Autodesk Fusion 360 part; units mm, degrees
(part 2 of 2)
sketch "Dovetail" plane through (75.5, 0, 0) normal (1, 0, 0) x (0, 1, 0)
  line L0 (-30.5, 0) -> (30.5, 0)
  line L1 (30.5, 0) -> (30.5, 32)
  line L2 (30.5, 32) -> (-30.5, 32)
  line L3 (-30.5, 32) -> (-30.5, 0)
  line L4 (-27.5, 32) -> (-27.5, 5.5)
  line L5 (-27.5, 5.5) -> (-27.5, 32)
  line L6 (27.5, 5.5) -> (27.5, 32)
  line L7 (27.5, 32) -> (27.5, 5.5)
  line L8 (30.5, 0) -> (30.5, 32)
  line L9 (-30.5, 0) -> (-30.5, 32)
  line L10 (-30.5, 29) -> (30.5, 29)
  line L11 (-28.9434, 29) -> (-27.5, 31.5)
  line L12 (-28.9434, 29) -> (-27.5, 29) construction
  line L13 (0, 2.5) -> (0, 20)
  line L14 (28.9434, 29) -> (27.5, 31.5)
  dimension "d19" = 3
  dimension "d20" = 60
  dimension "d21" = 0.5
  constraint coincident L9 L10.start
  constraint coincident L8 L10.end
  constraint perpendicular L8 L10
  constraint horizontal L12
  constraint coincident L10 L11.start
  constraint coincident L5 L11.end
  constraint symmetric L11.start L13 L14.start
  constraint symmetric L11.end L13 L14.end
  constraint coincident L4 L12.end
  measures "d19" distance of L2 L10
  measures "d20" angle of L11 L12
  measures "d21" distance of L2 L11.end
extrude "Extrude4" cut sketch "Dovetail" against normal up to surface (148 mm away) contours L4 L5 L10 L11 | L6 L7 L10 L14 | L2 L4 L5 L6 L7 L10 bodies 1
sketch "Lid" plane through (75.5, 0, 0) normal (1, 0, 0) x (0, 1, 0) in component "Lid"
  line L0 (27.5, 32) -> (27.5, 31.5)
  line L1 (27.5, 31.5) -> (28.9434, 29)
  line L2 (28.9434, 29) -> (-28.9434, 29)
  line L3 (-28.9434, 29) -> (-27.5, 31.5)
  line L4 (-27.5, 31.5) -> (-27.5, 32)
  line L5 (-27.5, 32) -> (-30.5, 32)
  line L6 (-30.5, 32) -> (-30.5, 0)
  line L7 (-30.5, 0) -> (30.5, 0)
  line L8 (30.5, 0) -> (30.5, 32)
  line L9 (30.5, 32) -> (27.5, 32)
  line L10 (-27.5, 31.5) -> (-27.2113, 32)
  line L11 (27.5, 31.5) -> (27.2113, 32)
  line L12 (-27.2113, 32) -> (27.2113, 32)
  constraint coincident L3.end L4.start
  constraint parallel L3 L10
  constraint coincident L0.end L1.start
  constraint parallel L1 L11
  constraint horizontal L12
  constraint collinear L5 L12
extrude "Extrude1'" add sketch "Lid" against normal up to surface (148 mm away) separate body contours L1 L2 L3 L10 L11 L12 makes body 2 in component "Lid"
move_face "OffsetFaces2" offset -0.5 4 faces at (-23.1667, 27.9811, 30.6667) (-23.1667, 27.4038, 31.6667) (-23.1667, -28.4623, 29.8333) (26.1667, -27.4038, 31.6667) on bodies 2 in component "Lid"
sketch "Top" plane through (0, 0, 32) normal (0, 0, 1) x (-1, 0, 0) in component "Lid"
  line L0 (72.5, -26.634) -> (72.5, 26.634)
  line L1 (72.5, 26.634) -> (-75.5, 26.634)
  line L2 (-75.5, 26.634) -> (-75.5, -26.634)
  line L3 (-75.5, -26.634) -> (72.5, -26.634)
  line L4 (-35.5, -15) -> (-50.5, -15)
  line L5 (-50.5, -15) -> (-50.5, 15)
  line L6 (-50.5, 15) -> (-35.5, 15)
  line L7 (-35.5, 15) -> (-35.5, -15)
  line L8 (-43, 15) -> (-43, 26.634) construction
  line L9 (-43, -15) -> (-43, -26.634) construction
  line L10 (-8.6603, -15) -> (8.6603, -15)
  line L11 (8.6603, -15) -> (17.3205, 0)
  line L12 (17.3205, 0) -> (8.6603, 15)
  line L13 (8.6603, 15) -> (-8.6603, 15)
  line L14 (-8.6603, 15) -> (-17.3205, 0)
  line L15 (-17.3205, 0) -> (-8.6603, -15)
  line L16 (72.5, 0) -> (0, 0) construction
  line L17 (0, 0) -> (0, -26.634) construction
  line L18 (-8.6603, -15) -> (17.3205, 0) construction
  line L19 (-17.3205, 0) -> (8.6603, 15) construction
  line L20 (8.6603, -15) -> (-8.6603, 15) construction
  dimension "d28" = 15
  dimension "d29" = 30
  dimension "d30" = 25
  dimension "d32" = 15
  constraint horizontal L4
  constraint vertical L5
  constraint horizontal L6
  constraint vertical L7
  constraint midpoint L6 L8.start
  constraint coincident L1 L8.end
  constraint perpendicular L1 L8
  constraint midpoint L4 L9.start
  constraint coincident L3 L9.end
  constraint perpendicular L3 L9
  constraint equal L8 L9
  constraint parallel L3 L10
  constraint midpoint L0 L16.start
  constraint coincident L16.end L17.start
  constraint coincident L3 L17.end
  constraint perpendicular L3 L17
  constraint coincident L17.start L16
  measures "d28" distance of L4.start L4.end
  measures "d29" distance of L4.start L6.end
  measures "d30" distance of L2 L5
  measures "d32" distance of L16.end L15
extrude "Extrude2'" cut sketch "Top" against normal up to surface (3 mm away) contours L10 L11 L12 L13 L14 L15 bodies 2 in component "Lid"
extrude "Extrude3'" add sketch "Top" along normal blind 2 contours L4 L5 L6 L7 bodies 2 in component "Lid"
copy_body "Body->Comp1" bodies 1 removing the originals makes body 3 in component "Base"
sketch "Mounting" plane through (0, -30.5, 0) normal (0, -1, 0) x (1, 0, 0) in component "Base"
  line L0 (-75.5, 0) -> (75.5, 0)
  line L1 (75.5, 0) -> (75.5, 32)
  line L2 (75.5, 32) -> (-75.5, 32)
  line L3 (-75.5, 32) -> (-75.5, 0)
  line L4 (-75.5, 24.5) -> (75.5, 24.5)
  line L5 (75.5, 24.5) -> (75.5, 19.5)
  line L6 (75.5, 19.5) -> (-75.5, 19.5)
  line L7 (-75.5, 24.5) -> (-75.5, 19.5)
  dimension "d38" = 5
  dimension "d39" = 7.5
  constraint coincident L3 L4.start
  constraint coincident L1 L4.end
  constraint perpendicular L1 L4
  constraint perpendicular L4 L5
  constraint coincident L3 L6.end
  constraint perpendicular L3 L6
  measures "d38" distance of L4.end L5.end
  measures "d39" distance of L2 L4
extrude "Extrude1''" add sketch "Mounting" along normal blind 7.5 separate body contours L1 L3 L4 L5 L6 L7 makes body 4 in component "Base"
sketch "ScrewHoles" plane through (0, 0, 24.5) normal (0, 0, 1) x (-1, 0, 0) in component "Base"
  line L0 (75.5, 30.5) -> (75.5, 38)
  line L1 (75.5, 38) -> (-75.5, 38)
  line L2 (-75.5, 38) -> (-75.5, 30.5)
  circle A0 centre (37.75, 34.25) radius 1.55
  circle A1 centre (-37.75, 34.25) radius 1.55
  line L3 (75.5, 38) -> (0, 30.5) construction
  line L4 (75.5, 30.5) -> (0, 38) construction
  line L5 (-75.5, 38) -> (0, 30.5) construction
  line L6 (0, 38) -> (-75.5, 30.5) construction
  line L7 (-75.5, 30.5) -> (75.5, 30.5)
  line L8 (0, 30.5) -> (0, 38) construction
  dimension "d42" = 3.1
  dimension "d43" = 3.1
  constraint coincident L0.end L1.start
  constraint coincident L0.start L4.start
  constraint midpoint L1 L4.end
  constraint coincident L1.end L2.start
  constraint coincident L2.end L6.end
  constraint coincident A1.centre L5
  constraint coincident A1.centre L6
  constraint coincident A0.centre L4
  constraint coincident A0.centre L3
  constraint perpendicular L1 L8
  constraint equal L3 L4
  measures "d42" diameter of A0
  measures "d43" diameter of A1
extrude "Extrude2''" cut sketch "ScrewHoles" against normal up to surface (5 mm away) contours A0 | A1 bodies 3 4 in component "Base"
sketch "Suport" plane through (-75.5, 0, 0) normal (-1, 0, 0) x (0, -1, 0) in component "Base"
  line L0 (30.5, 24.5) -> (30.5, 19.5)
  line L1 (30.5, 19.5) -> (38, 19.5)
  line L2 (38, 19.5) -> (38, 24.5)
  line L3 (38, 24.5) -> (30.5, 24.5)
  line L4 (30.5, 0) -> (30.5, 32)
  line L5 (30.5, 24.5) -> (38, 24.5)
  line L6 (30.5, 32) -> (38, 24.5)
  constraint coincident L4.end L6.start
  constraint coincident L2.end L3.start
extrude "Extrude3''" add sketch "Suport" against normal blind 5 separate body contours L3 L4 L5 L6 makes body 5 in component "Base"
mirror "Mirror1" about plane through (0, 0, 0) normal (1, 0, 0) of bodies 5 makes body 6 in component "Base"
combine "Combine1" operation add target body 4 tool bodies 6 5 in component "Base"
mirror "Mirror2" about plane through (0, 0, 0) normal (0, 1, 0) of bodies 4 makes body 7 in component "Base"
combine "Combine2" operation add target body 3 tool bodies 7 4 in component "Base"
component "Lid" placed x (1, 0, 0) y (0, 1, 0) z (0, 0, 1) at (0, 0, 0)
component "Base" placed x (1, 0, 0) y (0, 1, 0) z (0, 0, 1) at (0, 0, 0)
equation "Length = 145 mm"
equation "width = 55 mm"
equation "height = 25 mm"
equation "PrintThickness = 3 mm"
equation "d5 = Length"
equation "d6 = width"
equation "d7 = PrintThickness"
equation "d8 = PrintThickness"
equation "d10 = height + PrintThickness * 2 + 1 mm"
